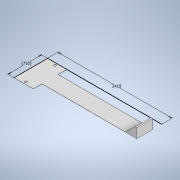
# Autodesk Inventor part: soporte
Saved by Autodesk Inventor 2021 (Build 250183000, 183)
## iProperties
Created: 2024-01-19
Part Number: soporte
Material: Generic
Document SubType Name: Modeling
Designer: MARCO BRAVO
Density: 1 g/cm^3
Appearance: Default
Author: MARCO BRAVO
Autodesk Inventor part; units mm, degrees
ref_plane "YZ Plane" through (0, 0, 0) normal (1, 0, 0) x (0, 1, 0)
ref_plane "XZ Plane" through (0, 0, 0) normal (0, 1, 0) x (-1, 0, 0)
ref_plane "XY Plane" through (0, 0, 0) normal (0, 0, 1) x (1, 0, 0)
sketch "Sketch1" plane through (0, 0, 0) normal (0, 1, 0) x (-1, 0, 0)
  line L0 (-266.0977, 629.1478) -> (143.9023, 629.1478)
  line L1 (143.9023, 629.1478) -> (143.9023, -80.8522)
  line L2 (143.9023, -80.8522) -> (-266.0977, -80.8522)
  line L3 (-266.0977, -80.8522) -> (-266.0977, 629.1478)
  circle A0 centre (-61.0977, 579.1478) radius 25
  circle A1 centre (-61.0977, -30.8522) radius 25
  point P0 (0, 0)
  dimension "d0" = 710
  dimension "d1" = 410
  dimension "d4" = 50
  dimension "d5" = 50
  constraints: 8 end point, 2 centre point, 2 parallel, 1 horizontal, 1 perpendicular
  measures "d0" distance of L0.end L1.end
  measures "d1" distance of L1.end L2.end
  measures "d4" diameter of A0
  measures "d5" diameter of A1
extrude "Extrusion1" add sketch "Sketch1" along normal blind 3
sketch "Sketch2" plane through (266.0977, 0, 629.1478) normal (1, 0, 0) x (0, 0, -1)
  line L0 (710, 3) -> (0, 3) projected
  line L1 (710, 3) -> (0, 3)
  line L2 (0, 3) -> (0, 0)
  line L3 (0, 0) -> (710, 0)
  line L4 (710, 0) -> (710, 3)
  line L5 (355, 0) -> (525, 0)
  line L6 (710, 0) -> (0, 0) projected
  line L7 (355, 3) -> (185, 3)
  line L8 (185, 3) -> (525, 3)
  line L9 (525, 3) -> (525, 0)
  line L10 (525, 0) -> (185, 0)
  line L11 (185, 0) -> (185, 3)
  point P0 (629.1478, 0)
  dimension "d8" = 170
  dimension "d9" = 170
  constraints: 20 end point, 4 perpendicular, 3 equal length, 2 midpoint, 2 point on line, 1 horizontal
  measures "d8" distance of L5.start L5.end
  measures "d9" distance of L7.start L7.end
extrude "Extrusion2" add sketch "Sketch2" along normal blind 2000 contours L9 L3 L11 L0
sketch "Sketch3" plane through (0, 3, 0) normal (0, 1, 0) x (1, 0, 0)
  line L0 (2266.0977, -104.1478) -> (2266.0977, -444.1478) projected
  line L1 (266.0977, -104.1478) -> (2266.0977, -104.1478) projected
  line L2 (2266.0977, -444.1478) -> (2236.0977, -444.1478)
  line L3 (2236.0977, -444.1478) -> (2236.0977, -104.1478)
  line L4 (2236.0977, -104.1478) -> (2266.0977, -104.1478)
  line L5 (2266.0977, -104.1478) -> (2266.0977, -444.1478)
  point P0 (0, 0)
  dimension "d12" = 340
  dimension "d13" = 30
  constraints: 8 end point, 2 parallel, 1 horizontal, 1 perpendicular, 1 point on line
  measures "d12" distance of L0.start L0.end
  measures "d13" distance of L0.end L2.end
extrude "Extrusion3" add sketch "Sketch3" along normal blind 200
sketch "Sketch4" plane through (266.0977, 0, 444.1478) normal (0, 0, 1) x (1, 0, 0)
  line L0 (1970, 3) -> (1970, 203) projected
  line L1 (1970, 203) -> (1970, 2.607)
  line L2 (0, 0) -> (2000, 0) projected
  line L3 (1970, 203) -> (1758.8495, 2.607)
  line L4 (1758.8495, 2.607) -> (1970, 2.607)
  line L5 (1970, 203) -> (1970, 2.607)
  point P0 (-266.0977, 0)
  constraints: 8 end point, 2 perpendicular, 1 horizontal
extrude "Extrusion4" add sketch "Sketch4" against normal blind 30
sketch "Sketch5" plane through (0, 3, 0) normal (0, 1, 0) x (1, 0, 0)
  line L0 (266.0977, 80.8522) -> (-143.9023, 80.8522) projected
  line L1 (-143.9023, 80.8522) -> (2266.0977, 80.8522)
  line L2 (-143.9023, 80.8522) -> (-143.9023, -629.1478) projected
  line L3 (-143.9023, 80.8522) -> (-143.9023, -629.1478)
  point P0 (0, 0)
  dimension "d18" = 2410
  dimension "d19" = 710
  constraints: 4 end point, 1 horizontal, 1 vertical
  measures "d18" distance of L0.end L1.end
  measures "d19" distance of L0.end L2.end
body "Solid1"
